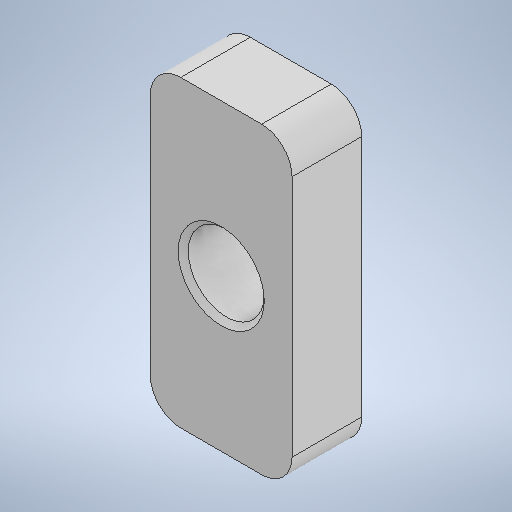
# Autodesk Inventor part: rapoukServoWasherv0
Saved by Autodesk Inventor 2025 (Build 290162000, 162)
## iProperties
Created: 2025-01-28
Part Number: rapoukServoWasherv0
Material: Všeobecné
Document SubType Name: Modeling
Designer: s21suk
Density: 1 g/cm^3
Appearance: Výchozí
Author: s21suk
## iProperties of the stored document rapoukServoWasherv0_3D tisk.ipt
Created: 2025-01-28
Part Number: rapoukServoWasherv0_3D tisk
Material: Všeobecné
Document SubType Name: Modeling
Designer: s21suk
Density: 1 g/cm^3
Appearance: Výchozí
Author: s21suk
Autodesk Inventor part; units mm, degrees
ref_plane "YZ Plane" through (0, 0, 0) normal (1, 0, 0) x (0, 1, 0)
ref_plane "XZ Plane" through (0, 0, 0) normal (0, 1, 0) x (-1, 0, 0)
ref_plane "XY Plane" through (0, 0, 0) normal (0, 0, 1) x (1, 0, 0)
sketch "Náčrt2" plane through (0, 0, 0) normal (0, 0, 1) x (1, 0, 0)
  line L0 (-2.8, -6) -> (2.8, -6)
  line L1 (2.8, -6) -> (2.8, 6)
  line L2 (2.8, 6) -> (-2.8, 6)
  line L3 (-2.8, 6) -> (-2.8, -6)
  line L4 (-2.8, -6) -> (2.8, 6) construction
  line L5 (2.8, -6) -> (-2.8, 6) construction
  circle A0 centre (0, 0) radius 1.5
  dimension "d0" = 5.6
  dimension "d1" = 12
  dimension "d2" = 3
  constraints: 12 end point, 2 midpoint, 2 parallel, 1 centre point, 1 coincident, 1 horizontal, 1 perpendicular
  measures "d0" distance of L2.end L1.end
  measures "d1" distance of L1.end L0.end
  measures "d2" diameter of A0
extrude "Vysunutí1" add sketch "Náčrt2" along normal blind 2.75
fillet "Zaoblení1" radius 1.2 4 edges at (-2.8, 6, 1.375) (2.8, 6, 1.375) (2.8, -6, 1.375) (-2.8, -6, 1.375)
chamfer "Zkosení1" distance 0.2 angle 45 2 edges at (-1.5, 0, 2.75) (-1.5, 0, 0)
